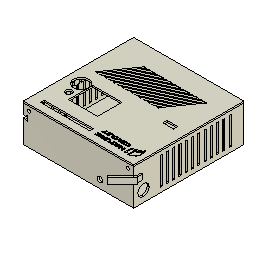
Focus maintainer v24 (Autodesk Fusion 360 design; units mm, degrees)
Autodesk Fusion 360 part; units mm, degrees
sketch "Sketch1" plane through (0, 0, 0) normal (0, 0, 1) x (1, 0, 0)
  line L0 (0, 0) -> (104, 0)
  line L1 (104, 0) -> (104, 104)
  line L2 (104, 104) -> (0, 104)
  line L3 (0, 104) -> (0, 0)
  line L4 (102.2, 1.8) -> (102.2, 102.2)
  line L5 (102.2, 102.2) -> (1.8, 102.2)
  line L6 (1.8, 102.2) -> (1.8, 1.8)
  line L7 (1.8, 1.8) -> (102.2, 1.8)
  dimension "d1" = 104
  dimension "d2" = 104
  dimension "d3" = -1.8
  constraint horizontal L0
  constraint vertical L1
  constraint horizontal L2
  constraint vertical L3
  constraint coincident L0.start L3.end
  measures "d1" distance of L0.start L0.end
  measures "d2" distance of L0.start L2.end
extrude "Extrude1" add sketch "Sketch1" against normal blind 1.5 contours L0 L1 L2 L3 | L4 L5 L6 L7 makes body 1
extrude "Extrude2" add sketch "Sketch1" along normal blind 32.5 bodies 1
hole "Hole1" at (5.5, 0, 28.5) direction (0, 1, 0) diameter 3 depth 105 tip angle 118 bodies 1
pattern_linear "R-Pattern1" count 2 spacing 93 along (1, 0, 0) of "Hole1"
sketch "Sketch2" plane through (0, 0, 0) normal (0, 0, 1) x (1, 0, 0)
  line L0 (0, 0) -> (104, 0)
  line L1 (104, 0) -> (104, 104)
  line L2 (104, 104) -> (0, 104)
  line L3 (0, 104) -> (0, 0)
  line L4 (102, 2) -> (102, 102)
  line L5 (102, 102) -> (2, 102)
  line L6 (2, 102) -> (2, 2)
  line L7 (2, 2) -> (102, 2)
  line L8 (100, 4) -> (100, 100)
  line L9 (100, 100) -> (4, 100)
  line L10 (4, 100) -> (4, 4)
  line L11 (4, 4) -> (100, 4)
  dimension "d17" = 104
  dimension "d18" = 104
  dimension "d19" = -2
  dimension "d20" = -4
  constraint horizontal L0
  constraint vertical L1
  constraint horizontal L2
  constraint vertical L3
  constraint coincident L0.start L3.end
  measures "d17" distance of L0.start L0.end
  measures "d18" distance of L0.start L2.end
extrude "Extrude3" add sketch "Sketch1" sketch "Sketch2" against normal blind 1.5 separate body contours L0 L1 L2 L3 | L4 L5 L6 L7 of sketch 2 contours L0 L1 L2 L3 | L4 L5 L6 L7 | L8 L9 L10 L11 makes body 2
extrude "Extrude4" add sketch "Sketch2" along normal blind 6.5 contours L4 L5 L6 L7 bodies 2
hole "Hole2" at (5.5, 2, 4.1) direction (0, 1, 0) diameter 3 depth 110 tip angle 118 bodies 2
pattern_linear "R-Pattern2" count 2 spacing 93 along (1, 0, 0) of "Hole2"
sketch "Sketch3" plane through (0, 0, 0) normal (0, 0, 1) x (1, 0, 0)
  line L0 (20, 81.5) -> (47.5, 81.5)
  line L1 (47.5, 81.5) -> (47.5, 58.5)
  line L2 (47.5, 58.5) -> (20, 58.5)
  line L3 (20, 58.5) -> (20, 81.5)
  line L4 (100, 100) -> (4, 100)
  line L5 (100, 4) -> (100, 100)
  circle A0 centre (12.9, 62.5) radius 7.1
  line L6 (9, 97) -> (55.5, 97)
  line L7 (55.5, 97) -> (55.5, 93.5)
  line L8 (55.5, 93.5) -> (9, 93.5)
  line L9 (9, 93.5) -> (9, 97)
  circle A1 centre (14, 75) radius 3
  line L10 (4, 4) -> (4, 100)
  line L11 (83.5, 56) -> (93.5, 56)
  line L12 (93.5, 56) -> (93.5, 52)
  line L13 (93.5, 52) -> (83.5, 52)
  line L14 (83.5, 52) -> (83.5, 56)
  line L15 (31, 19) -> (29, 19)
  line L16 (29, 19) -> (10.072, 46.032)
  line L17 (31, 19) -> (12.0419, 46.032)
  line L18 (12.0419, 46.032) -> (10.072, 46.032)
  line L19 (35.0714, 19) -> (33.0714, 19)
  line L20 (33.0714, 19) -> (14.1434, 46.032)
  line L21 (35.0714, 19) -> (16.1133, 46.032)
  line L22 (16.1133, 46.032) -> (14.1434, 46.032)
  line L23 (39.1429, 19) -> (37.1429, 19)
  line L24 (37.1429, 19) -> (18.2148, 46.032)
  line L25 (39.1429, 19) -> (20.1847, 46.032)
  line L26 (20.1847, 46.032) -> (18.2148, 46.032)
  line L27 (43.2143, 19) -> (41.2143, 19)
  line L28 (41.2143, 19) -> (22.2863, 46.032)
  line L29 (43.2143, 19) -> (24.2561, 46.032)
  line L30 (24.2561, 46.032) -> (22.2863, 46.032)
  line L31 (47.2857, 19) -> (45.2857, 19)
  line L32 (45.2857, 19) -> (26.3577, 46.032)
  line L33 (47.2857, 19) -> (28.3276, 46.032)
  line L34 (28.3276, 46.032) -> (26.3577, 46.032)
  line L35 (51.3571, 19) -> (49.3571, 19)
  line L36 (49.3571, 19) -> (30.4291, 46.032)
  line L37 (51.3571, 19) -> (32.399, 46.032)
  line L38 (32.399, 46.032) -> (30.4291, 46.032)
  line L39 (55.4286, 19) -> (53.4286, 19)
  line L40 (53.4286, 19) -> (34.5005, 46.032)
  line L41 (55.4286, 19) -> (36.4704, 46.032)
  line L42 (36.4704, 46.032) -> (34.5005, 46.032)
  line L43 (59.5, 19) -> (57.5, 19)
  line L44 (57.5, 19) -> (38.572, 46.032)
  line L45 (59.5, 19) -> (40.5419, 46.032)
  line L46 (40.5419, 46.032) -> (38.572, 46.032)
  line L47 (63.5714, 19) -> (61.5714, 19)
  line L48 (61.5714, 19) -> (42.6434, 46.032)
  line L49 (63.5714, 19) -> (44.6133, 46.032)
  line L50 (44.6133, 46.032) -> (42.6434, 46.032)
  line L51 (67.6429, 19) -> (65.6429, 19)
  line L52 (65.6429, 19) -> (46.7148, 46.032)
  line L53 (67.6429, 19) -> (48.6847, 46.032)
  line L54 (48.6847, 46.032) -> (46.7148, 46.032)
  line L55 (71.7143, 19) -> (69.7143, 19)
  line L56 (69.7143, 19) -> (50.7863, 46.032)
  line L57 (71.7143, 19) -> (52.7561, 46.032)
  line L58 (52.7561, 46.032) -> (50.7863, 46.032)
  line L59 (75.7857, 19) -> (73.7857, 19)
  line L60 (73.7857, 19) -> (54.8577, 46.032)
  line L61 (75.7857, 19) -> (56.8276, 46.032)
  line L62 (56.8276, 46.032) -> (54.8577, 46.032)
  line L63 (79.8571, 19) -> (77.8571, 19)
  line L64 (77.8571, 19) -> (58.9291, 46.032)
  line L65 (79.8571, 19) -> (60.899, 46.032)
  line L66 (60.899, 46.032) -> (58.9291, 46.032)
  line L67 (83.9286, 19) -> (81.9286, 19)
  line L68 (81.9286, 19) -> (63.0005, 46.032)
  line L69 (83.9286, 19) -> (64.9704, 46.032)
  line L70 (64.9704, 46.032) -> (63.0005, 46.032)
  line L71 (88, 19) -> (86, 19)
  line L72 (86, 19) -> (67.072, 46.032)
  line L73 (88, 19) -> (69.0419, 46.032)
  line L74 (69.0419, 46.032) -> (67.072, 46.032)
  dimension "d34" = 18.5
  dimension "d36" = 27.5
  dimension "d37" = 23
  dimension "d38" = 14.2
  dimension "d39" = 19
  dimension "d41" = 3
  dimension "d42" = 46.5
  dimension "d43" = 3.5
  dimension "d44" = 6
  dimension "d45" = 25
  dimension "d48" = 16
  dimension "d50" = 7.1
  dimension "d51" = 10
  dimension "d52" = 5
  dimension "d53" = 44
  dimension "d54" = 6.5
  dimension "d55" = 10
  dimension "d56" = 4
  dimension "d63" = 33
  dimension "d68" = 15
  dimension "d71" = 57
  dimension "d72" = 0
  constraint horizontal L0
  constraint vertical L1
  constraint horizontal L2
  constraint vertical L3
  constraint horizontal L6
  constraint vertical L7
  constraint horizontal L8
  constraint vertical L9
  constraint horizontal L11
  constraint vertical L12
  constraint horizontal L13
  constraint vertical L14
  constraint horizontal L15
  constraint parallel L15 L18
  measures "d34" distance of L0.end L4
  measures "d36" distance of L0.start L0.end
  measures "d37" distance of L0.start L2.end
  measures "d38" diameter of A0
  measures "d39" vertical distance of L0.end A0.centre
  measures "d41" distance of L4 L6.end
  measures "d42" distance of L7.end L8.end
  measures "d43" distance of L6.start L8.end
  measures "d44" diameter of A1
  measures "d45" vertical distance of L4.start A1.centre
  measures "d48" horizontal distance of L0.start L4.end
  measures "d50" horizontal distance of L2.end A0.centre
  measures "d51" distance of A1.centre L10
  measures "d52" horizontal distance of L6.start L4.end
  measures "d53" vertical distance of L4.start L11.end
  measures "d54" horizontal distance of L4.start L11.end
  measures "d55" distance of L12.end L13.end
  measures "d56" distance of L11.start L13.end
  measures "d63" distance of L15.end L16.end
  measures "d68" distance of L10.start L15
extrude "Extrude5" cut sketch "Sketch3" against normal blind 1.5 bodies 2
sketch "Sketch4" plane through (102.2, 0, 0) normal (-1, 0, 0) x (0, -1, 0)
  line L0 (-102.2, 0) -> (-1.8, 0)
  line L1 (-1.8, 0) -> (-1.8, 32.5)
  line L2 (-1.8, 32.5) -> (-102.2, 32.5)
  line L3 (-102.2, 32.5) -> (-102.2, 0)
  line L4 (-6.8, 3.5) -> (-10.8544, 3.5)
  line L5 (-4.05, 3.5) -> (-14.55, 3.5)
  line L6 (-14.55, 3.5) -> (-14.55, 14)
  line L7 (-14.55, 14) -> (-4.05, 14)
  line L8 (-4.05, 14) -> (-4.05, 3.5)
  dimension "d86" = 10.5
  dimension "d87" = 10.5
  dimension "d88" = 2.25
  dimension "d89" = 3.5
  constraint horizontal L4
  constraint horizontal L5
  constraint vertical L6
  constraint horizontal L7
  constraint vertical L8
  measures "d86" distance of L5.start L5.end
  measures "d87" distance of L5.start L7.end
  measures "d88" distance of L1 L5.start
  measures "d89" distance of L0 L5
sketch "Sketch5" plane through (0, 1.8, 0) normal (0, 1, 0) x (-1, 0, 0)
  circle A0 centre (-98.5, 28.5) radius 1.5
  circle A1 centre (-5.5, 28.5) radius 1.5
  line L0 (-102.2, 0) -> (-1.8, 0)
  line L1 (-1.8, 0) -> (-1.8, 32.5)
  line L2 (-1.8, 32.5) -> (-102.2, 32.5)
  line L3 (-102.2, 32.5) -> (-102.2, 0)
  circle A2 centre (-72.2, 6) radius 2.5
  dimension "d79" = 5
  dimension "d80" = 30
  dimension "d81" = 6
  measures "d79" diameter of A2
  measures "d80" distance of L3 A2.centre
  measures "d81" distance of L0 A2.centre
extrude "Extrude7" cut sketch "Sketch5" against normal blind 6 contours A2 bodies 1
extrude "Extrude8" cut sketch "Sketch4" against normal blind 2 contours L4 L5 L6 L7 L8 bodies 1
fillet "Fillet1" radius 5 4 edges at (103.1, 4.05, 14) (103.1, 14.55, 14) (103.1, 14.55, 3.5) (103.1, 4.05, 3.5) on bodies 1
sketch "Sketch6" plane through (0, 0, 0) normal (0, -1, 0) x (1, 0, 0)
  circle A0 centre (72.2, 6) radius 2.5
  circle A1 centre (98.5, 28.5) radius 1.5
  circle A2 centre (5.5, 28.5) radius 1.5
  line L0 (0, 32.5) -> (0, -1.5)
  line L1 (0, -1.5) -> (104, -1.5)
  line L2 (104, -1.5) -> (104, 32.5)
  line L3 (104, 32.5) -> (0, 32.5)
  line L4 (104, 22.7437) -> (102, 22.7437)
  line L5 (102, 22.7437) -> (100.4679, 24.0293)
  line L6 (100.4679, 24.0293) -> (100.4679, 19.0293)
  line L7 (100.4679, 19.0293) -> (102, 20.3149)
  line L8 (100.4679, 19.0293) -> (102.4679, 19.0293) construction
  line L9 (102, 20.3149) -> (104, 20.3149)
  line L10 (104, 20.3149) -> (104, 22.7437)
  line L11 (52, -1.5) -> (52, 32.5)
  line L12 (2, 22.7437) -> (3.5321, 24.0293)
  line L13 (3.5321, 24.0293) -> (3.5321, 19.0293)
  line L14 (3.5321, 19.0293) -> (1.5321, 19.0293) construction
  line L15 (3.5321, 19.0293) -> (2, 20.3149)
  line L16 (0, 22.7437) -> (2, 22.7437)
  line L17 (2, 20.3149) -> (0, 20.3149)
  line L18 (104, 22.7437) -> (104.2, 22.7437)
  line L19 (104.2, 22.7437) -> (104.2, 23.9437)
  line L20 (104.2, 23.9437) -> (105.7, 23.9437)
  line L21 (104, 20.3149) -> (104.2, 20.3149)
  line L22 (104.2, 20.3149) -> (104.2, 19.1149)
  line L23 (104.2, 19.1149) -> (105.7, 19.1149)
  line L24 (105.7, 19.1149) -> (105.7, 23.9437)
  dimension "d92" = 2
  dimension "d93" = 140
  dimension "d94" = 2
  dimension "d95" = 5
  dimension "d96" = 2
  dimension "d97" = 40
  dimension "d129" = 0.2
  dimension "d130" = 1.2
  dimension "d131" = 1.5
  dimension "d132" = 0.2
  dimension "d133" = 1.2
  dimension "d134" = 1.5
  constraint coincident L2 L4.start
  constraint perpendicular L2 L4
  constraint vertical L6
  constraint horizontal L8
  constraint coincident L2 L9.end
  constraint perpendicular L2 L9
  constraint midpoint L1 L11.start
  constraint midpoint L3 L11.end
  constraint symmetric L4.start L11 L16.start
  constraint symmetric L4.end L11 L12.start
  constraint symmetric L5.end L11 L12.end
  constraint symmetric L6.end L11 L13.end
  constraint symmetric L7.end L11 L15.end
  constraint symmetric L8.end L11 L14.end
  constraint symmetric L9.end L11 L17.end
  constraint perpendicular L2 L18
  constraint perpendicular L4 L19
  constraint perpendicular L19 L20
  constraint perpendicular L2 L21
  constraint perpendicular L21 L22
  constraint perpendicular L22 L23
  measures "d92" distance of L4.start L4.end
  measures "d93" angle of L4 L5
  measures "d94" distance of L4.end L5.end
  measures "d95" distance of L5.end L6.end
  measures "d96" distance of L6.end L7.end
  measures "d97" angle of L7 L8
  measures "d129" distance of L4.start L18.end
  measures "d130" distance of L18.end L19.end
  measures "d131" distance of L19.end L20.end
  measures "d132" distance of L9.end L21.end
  measures "d133" distance of L21.end L22.end
  measures "d134" distance of L22.end L23.end
extrude "Extrude9" cut sketch "Sketch6" against normal blind 7 contours L0 L12 L13 L15 L16 L17 | L2 L4 L5 L6 L7 L9 L10 bodies 1
extrude "Extrude10" add sketch "Sketch6" along normal blind -7 and the other way blind -8 separate body contours L2 L10 L18 L19 L20 L21 L22 L23 L24 | L2 L4 L5 L6 L7 L9 L10 makes body 3
ref_plane "WorkPlane1" through (104, 0, 21.5293) normal (-0.707107, 0.707107, 0) x (0, 0, 1)
sketch "Sketch7" plane through (52, -52, 0) normal (-0.707107, 0.707107, 0) x (0, 0, 1)
  line L0 (19, 76) -> (24.9317, 76)
  line L1 (24.9317, 76) -> (24.9317, 56)
  line L2 (24.9317, 56) -> (19, 56)
  line L3 (19, 56) -> (19, 76)
  dimension "d105" = 20
  constraint horizontal L0
  constraint vertical L1
  constraint horizontal L2
  constraint vertical L3
  measures "d105" distance of L0.start L2.end
extrude "Extrude11" cut sketch "Sketch7" against normal blind 8 bodies 3
extrude "Extrude12" add sketch "Sketch7" against normal blind 2 bodies 3
move_face "OffsetFaces1" offset -0.2 5 faces at (102.7333, 1.7333, 22.7437) (100.9786, 0.4893, 23.6008) (100.4679, -0.0214, 22.3626) (100.9786, 0.4893, 19.4578) (102.7333, 1.7333, 20.3149) on bodies 3
sketch "Sketch8" plane through (0, 0, 0) normal (-1, 0, 0) x (0, -1, 0)
  line L0 (-7, 22.7437) -> (0, 22.7437)
  line L1 (0, 22.7437) -> (0, 32.5)
  line L2 (0, 32.5) -> (-104, 32.5)
  line L3 (-104, 32.5) -> (-104, -1.5)
  line L4 (-104, -1.5) -> (0, -1.5)
  line L5 (0, -1.5) -> (0, 20.3149)
  line L6 (0, 20.3149) -> (-7, 20.3149)
  line L7 (-7, 20.3149) -> (-7, 22.7437)
  line L8 (-92, 29) -> (-90, 29)
  line L9 (-90, 29) -> (-90, 3)
  line L10 (-90, 3) -> (-92, 3)
  line L11 (-92, 3) -> (-92, 29)
  constraint horizontal L8
  constraint vertical L9
  constraint horizontal L10
  constraint vertical L11
extrude "Extrude13" cut sketch "Sketch8" against normal blind 120 contours L8 L9 L10 L11 bodies 1
pattern_linear "R-Pattern3" count 12 spacing 5.9091 along (0, -1, 0) of "Extrude13"
sketch "Sketch9" plane through (0, 0, -1.5) normal (0, 0, -1) x (1, 0, 0)
  line L0 (60.899, -46.032) -> (58.9291, -46.032)
  line L1 (58.9291, -46.032) -> (77.8571, -19)
  line L2 (77.8571, -19) -> (79.8571, -19)
  line L3 (79.8571, -19) -> (60.899, -46.032)
  line L4 (44.6133, -46.032) -> (42.6434, -46.032)
  line L5 (42.6434, -46.032) -> (61.5714, -19)
  line L6 (61.5714, -19) -> (63.5714, -19)
  line L7 (63.5714, -19) -> (44.6133, -46.032)
  line L8 (28.3276, -46.032) -> (26.3577, -46.032)
  line L9 (26.3577, -46.032) -> (45.2857, -19)
  line L10 (45.2857, -19) -> (47.2857, -19)
  line L11 (47.2857, -19) -> (28.3276, -46.032)
  line L12 (12.0419, -46.032) -> (10.072, -46.032)
  line L13 (10.072, -46.032) -> (29, -19)
  line L14 (29, -19) -> (31, -19)
  line L15 (31, -19) -> (12.0419, -46.032)
  circle A0 centre (14, -75) radius 3
  line L16 (16.1133, -46.032) -> (14.1434, -46.032)
  line L17 (14.1434, -46.032) -> (33.0714, -19)
  line L18 (33.0714, -19) -> (35.0714, -19)
  line L19 (35.0714, -19) -> (16.1133, -46.032)
  line L20 (32.399, -46.032) -> (30.4291, -46.032)
  line L21 (30.4291, -46.032) -> (49.3571, -19)
  line L22 (49.3571, -19) -> (51.3571, -19)
  line L23 (51.3571, -19) -> (32.399, -46.032)
  line L24 (48.6847, -46.032) -> (46.7148, -46.032)
  line L25 (46.7148, -46.032) -> (65.6429, -19)
  line L26 (65.6429, -19) -> (67.6429, -19)
  line L27 (67.6429, -19) -> (48.6847, -46.032)
  line L28 (64.9704, -46.032) -> (63.0005, -46.032)
  line L29 (63.0005, -46.032) -> (81.9286, -19)
  line L30 (81.9286, -19) -> (83.9286, -19)
  line L31 (83.9286, -19) -> (64.9704, -46.032)
  line L32 (56.8276, -46.032) -> (54.8577, -46.032)
  line L33 (54.8577, -46.032) -> (73.7857, -19)
  line L34 (73.7857, -19) -> (75.7857, -19)
  line L35 (75.7857, -19) -> (56.8276, -46.032)
  line L36 (40.5419, -46.032) -> (38.572, -46.032)
  line L37 (38.572, -46.032) -> (57.5, -19)
  line L38 (57.5, -19) -> (59.5, -19)
  line L39 (59.5, -19) -> (40.5419, -46.032)
  line L40 (24.2561, -46.032) -> (22.2863, -46.032)
  line L41 (22.2863, -46.032) -> (41.2143, -19)
  line L42 (41.2143, -19) -> (43.2143, -19)
  line L43 (43.2143, -19) -> (24.2561, -46.032)
  line L44 (93.5, -52) -> (93.5, -56)
  line L45 (93.5, -56) -> (83.5, -56)
  line L46 (83.5, -56) -> (83.5, -52)
  line L47 (83.5, -52) -> (93.5, -52)
  line L48 (47.5, -58.5) -> (47.5, -81.5)
  line L49 (47.5, -81.5) -> (20, -81.5)
  line L50 (20, -81.5) -> (20, -62.5)
  circle A1 centre (12.9, -62.5) radius 7.1
  line L51 (20, -62.5) -> (20, -58.5)
  line L52 (20, -58.5) -> (47.5, -58.5)
  line L53 (55.5, -93.5) -> (55.5, -97)
  line L54 (55.5, -97) -> (9, -97)
  line L55 (9, -97) -> (9, -93.5)
  line L56 (9, -93.5) -> (55.5, -93.5)
  line L57 (20.1847, -46.032) -> (18.2148, -46.032)
  line L58 (18.2148, -46.032) -> (37.1429, -19)
  line L59 (37.1429, -19) -> (39.1429, -19)
  line L60 (39.1429, -19) -> (20.1847, -46.032)
  line L61 (36.4704, -46.032) -> (34.5005, -46.032)
  line L62 (34.5005, -46.032) -> (53.4286, -19)
  line L63 (53.4286, -19) -> (55.4286, -19)
  line L64 (55.4286, -19) -> (36.4704, -46.032)
  line L65 (52.7561, -46.032) -> (50.7863, -46.032)
  line L66 (50.7863, -46.032) -> (69.7143, -19)
  line L67 (69.7143, -19) -> (71.7143, -19)
  line L68 (71.7143, -19) -> (52.7561, -46.032)
  line L69 (69.0419, -46.032) -> (67.072, -46.032)
  line L70 (67.072, -46.032) -> (86, -19)
  line L71 (86, -19) -> (88, -19)
  line L72 (88, -19) -> (69.0419, -46.032)
  line L73 (0, 0) -> (0, -104)
  line L74 (0, -104) -> (104, -104)
  line L75 (104, -104) -> (104, 0)
  line L76 (104, 0) -> (0, 0)
  spline S0 degree 3 poles (98.7844, -87.4951) (99.1077, -88.4839) (99.0819, -89.3983) (99.0819, -90.4193) knots 0 0 0 0 1 1 1 1
  spline S1 degree 3 poles (99.0819, -90.4193) (99.0819, -92.0513) (99.3129, -93.8226) (98.2772, -95.2143) knots 0 0 0 0 1 1 1 1
  spline S2 degree 3 poles (98.2772, -95.2143) (97.4381, -96.3429) (95.5453, -97.168) (94.2868, -97.8019) knots 0 0 0 0 1 1 1 1
  line L77 (94.2868, -97.8019) -> (92.7057, -98.6644)
  line L78 (92.7057, -98.6644) -> (92.7057, -97.8457)
  line L79 (92.7057, -97.8457) -> (92.6495, -97.144)
  line L80 (92.6495, -97.144) -> (92.6495, -96.957)
  line L81 (92.6495, -96.957) -> (92.6495, -96.5105)
  line L82 (92.6495, -96.5105) -> (92.6495, -94.9219)
  spline S3 degree 3 poles (92.6495, -94.9219) (92.6495, -94.0261) (92.6103, -93.2367) (93.1635, -92.4659) knots 0 0 0 0 1 1 1 1
  spline S4 degree 3 poles (93.1635, -92.4659) (93.5115, -91.9806) (94.0021, -91.7169) (94.5207, -91.4572) knots 0 0 0 0 1 1 1 1
  spline S5 degree 3 poles (94.5207, -91.4572) (95.4932, -90.9713) (96.7762, -90.6432) (97.62, -89.9795) knots 0 0 0 0 1 1 1 1
  spline S6 degree 3 poles (97.62, -89.9795) (98.1006, -89.6018) (98.4831, -89.1381) (98.6603, -88.548) knots 0 0 0 0 1 1 1 1
  line L83 (98.6603, -88.548) -> (98.7844, -87.4951)
  spline S7 degree 3 poles (89.3158, -98.1858) (89.2071, -97.9116) (89.2573, -97.0104) (89.2573, -96.6654) knots 0 0 0 0 1 1 1 1
  line L84 (89.2573, -96.6654) -> (89.2573, -93.8586)
  spline S8 degree 3 poles (89.2573, -93.8586) (89.2573, -93.1575) (89.1597, -92.7107) (89.6041, -92.1043) knots 0 0 0 0 1 1 1 1
  spline S9 degree 3 poles (89.6041, -92.1043) (90.2228, -91.2599) (91.7285, -90.6968) (92.7074, -90.3693) knots 0 0 0 0 1 1 1 1
  spline S10 degree 3 poles (92.7074, -90.3693) (93.957, -89.9512) (95.223, -89.5799) (96.3914, -88.9595) knots 0 0 0 0 1 1 1 1
  spline S11 degree 3 poles (96.3914, -88.9595) (97.4907, -88.3759) (98.0825, -87.7104) (97.8533, -86.4322) knots 0 0 0 0 1 1 1 1
  spline S12 degree 3 poles (97.8533, -86.4322) (98.2486, -86.6444) (98.745, -87.207) (98.8316, -87.6602) knots 0 0 0 0 1 1 1 1
  spline S13 degree 3 poles (98.8316, -87.6602) (98.9433, -88.2438) (98.5737, -89.0998) (98.1936, -89.5314) knots 0 0 0 0 1 1 1 1
  spline S14 degree 3 poles (98.1936, -89.5314) (96.9879, -90.9015) (94.6237, -90.998) (93.4144, -92.2803) knots 0 0 0 0 1 1 1 1
  spline S15 degree 3 poles (93.4144, -92.2803) (92.4829, -93.2686) (92.7097, -94.8188) (92.7074, -96.0807) knots 0 0 0 0 1 1 1 1
  spline S16 degree 3 poles (92.7074, -96.0807) (92.7074, -96.2035) (92.7221, -96.4087) (92.6495, -96.5105) knots 0 0 0 0 1 1 1 1
  spline S17 degree 3 poles (92.6495, -96.5105) (92.5583, -96.638) (91.9496, -96.8391) (91.7718, -96.9111) knots 0 0 0 0 1 1 1 1
  spline S18 degree 3 poles (91.7718, -96.9111) (90.9941, -97.2245) (89.9737, -97.6783) (89.3158, -98.1858) knots 0 0 0 0 1 1 1 1
  line L85 (86.7727, -97.3774) -> (86.2481, -97.3774)
  spline S19 degree 2 poles (86.2481, -97.3774) (85.9825, -97.3774) (85.7363, -97.1526) knots 0 0 0 1 1 1
  line L86 (85.7363, -97.1526) -> (83.7383, -95.5315)
  line L87 (83.7383, -95.5315) -> (83.7383, -97.0241)
  spline S20 degree 2 poles (83.7383, -97.0241) (83.7383, -97.2618) (83.4877, -97.3646) knots 0 0 0 1 1 1
  spline S21 degree 2 poles (83.4877, -97.3646) (83.4385, -97.3774) (83.3935, -97.3774) knots 0 0 0 1 1 1
  line L88 (83.3935, -97.3774) -> (82.8196, -97.3774)
  line L89 (82.8196, -97.3774) -> (82.8196, -94.3066)
  line L90 (82.8196, -94.3066) -> (83.3443, -94.3066)
  spline S22 degree 2 poles (83.3443, -94.3066) (83.6162, -94.3066) (83.8903, -94.5614) knots 0 0 0 1 1 1
  spline S23 degree 2 poles (83.8903, -94.5614) (83.8925, -94.5635) (84.0124, -94.6578) knots 0 0 0 1 1 1
  spline S24 degree 2 poles (84.0124, -94.6578) (84.1302, -94.752) (84.3721, -94.9447) knots 0 0 0 1 1 1
  spline S25 degree 2 poles (84.3721, -94.9447) (84.612, -95.1374) (84.9803, -95.4308) knots 0 0 0 1 1 1
  spline S26 degree 2 poles (84.9803, -95.4308) (85.3487, -95.7242) (85.8498, -96.1268) knots 0 0 0 1 1 1
  line L91 (85.8498, -96.1268) -> (85.854, -96.1268)
  line L92 (85.854, -96.1268) -> (85.854, -94.3066)
  line L93 (85.854, -94.3066) -> (86.7727, -94.3066)
  line L94 (86.7727, -94.3066) -> (86.7727, -97.3774)
  spline S27 degree 2 poles (80.3805, -94.4608) (80.3805, -94.5871) (80.3291, -94.7006) knots 0 0 0 1 1 1
  spline S28 degree 2 poles (80.3291, -94.7006) (80.2755, -94.8162) (80.1813, -94.904) knots 0 0 0 1 1 1
  spline S29 degree 2 poles (80.1813, -94.904) (80.0871, -94.994) (79.9586, -95.0454) knots 0 0 0 1 1 1
  spline S30 degree 2 poles (79.9586, -95.0454) (79.828, -95.0989) (79.6738, -95.0989) knots 0 0 0 1 1 1
  line L95 (79.6738, -95.0989) -> (78.9928, -95.0989)
  line L96 (78.9928, -95.0989) -> (79.8644, -96.5144)
  line L97 (79.8644, -96.5144) -> (81.2349, -94.2959)
  spline S31 degree 2 poles (81.2349, -94.2959) (82.2842, -94.2959) (82.2842, -94.298) knots 0 0 0 1 1 1
  spline S32 degree 2 poles (82.2842, -94.298) (82.2543, -94.3451) (82.1814, -94.4608) knots 0 0 0 1 1 1
  spline S33 degree 2 poles (82.1814, -94.4608) (82.1086, -94.5785) (82.0037, -94.7477) knots 0 0 0 1 1 1
  spline S34 degree 2 poles (82.0037, -94.7477) (81.8988, -94.9169) (81.7681, -95.1289) knots 0 0 0 1 1 1
  spline S35 degree 2 poles (81.7681, -95.1289) (81.6375, -95.343) (81.4919, -95.5807) knots 0 0 0 1 1 1
  spline S36 degree 2 poles (81.4919, -95.5807) (81.3441, -95.8184) (81.1878, -96.0711) knots 0 0 0 1 1 1
  spline S37 degree 2 poles (81.1878, -96.0711) (81.0315, -96.3238) (80.8773, -96.5744) knots 0 0 0 1 1 1
  spline S38 degree 2 poles (80.8773, -96.5744) (80.8023, -96.6986) (80.7424, -96.7949) knots 0 0 0 1 1 1
  spline S39 degree 2 poles (80.7424, -96.7949) (80.6824, -96.8934) (80.631, -96.9663) knots 0 0 0 1 1 1
  spline S40 degree 2 poles (80.631, -96.9663) (80.5796, -97.0391) (80.5368, -97.0883) knots 0 0 0 1 1 1
  spline S41 degree 2 poles (80.5368, -97.0883) (80.4918, -97.1397) (80.449, -97.1675) knots 0 0 0 1 1 1
  spline S42 degree 2 poles (80.449, -97.1675) (80.3077, -97.2768) (80.1621, -97.3217) knots 0 0 0 1 1 1
  spline S43 degree 2 poles (80.1621, -97.3217) (80.0143, -97.3667) (79.8323, -97.3667) knots 0 0 0 1 1 1
  spline S44 degree 2 poles (79.8323, -97.3667) (79.6781, -97.3667) (79.5132, -97.3003) knots 0 0 0 1 1 1
  spline S45 degree 2 poles (79.5132, -97.3003) (79.3483, -97.2339) (79.1813, -97.0669) knots 0 0 0 1 1 1
  spline S46 degree 2 poles (79.1813, -97.0669) (79.0935, -96.9705) (79.0571, -96.9063) knots 0 0 0 1 1 1
  line L98 (79.0571, -96.9063) -> (77.4467, -94.2959)
  line L99 (77.4467, -94.2959) -> (80.3783, -94.2959)
  line L100 (80.3783, -94.2959) -> (80.3805, -94.4608)
  line L101 (76.6329, -96.5422) -> (78.0506, -96.5422)
  line L102 (78.0506, -96.5422) -> (78.0506, -96.6729)
  spline S47 degree 2 poles (78.0506, -96.6729) (78.0506, -96.8977) (77.8536, -97.1333) knots 0 0 0 1 1 1
  spline S48 degree 2 poles (77.8536, -97.1333) (77.6715, -97.3025) (77.5538, -97.326) knots 0 0 0 1 1 1
  spline S49 degree 2 poles (77.5538, -97.326) (77.4467, -97.3667) (77.3567, -97.3667) knots 0 0 0 1 1 1
  line L103 (77.3567, -97.3667) -> (74.2859, -97.3667)
  line L104 (74.2859, -97.3667) -> (74.2859, -97.2404)
  spline S50 degree 2 poles (74.2859, -97.2404) (74.2859, -97.0134) (74.4786, -96.7842) knots 0 0 0 1 1 1
  spline S51 degree 2 poles (74.4786, -96.7842) (74.6757, -96.5422) (75.1146, -96.5422) knots 0 0 0 1 1 1
  line L105 (75.1146, -96.5422) -> (75.71, -96.5422)
  line L106 (75.71, -96.5422) -> (75.71, -94.2959)
  line L107 (75.71, -94.2959) -> (76.6329, -94.2959)
  line L108 (76.6329, -94.2959) -> (76.6329, -96.5422)
  spline S52 degree 2 poles (73.7505, -96.9877) (73.7505, -97.2318) (73.4764, -97.3517) knots 0 0 0 1 1 1
  spline S53 degree 2 poles (73.4764, -97.3517) (73.4293, -97.3667) (73.3715, -97.3667) knots 0 0 0 1 1 1
  line L109 (73.3715, -97.3667) -> (72.8554, -97.3667)
  line L110 (72.8554, -97.3667) -> (72.8554, -95.8377)
  spline S54 degree 2 poles (72.8554, -95.8377) (72.8554, -95.7049) (72.8147, -95.5979) knots 0 0 0 1 1 1
  spline S55 degree 2 poles (72.8147, -95.5979) (72.7719, -95.4908) (72.7012, -95.4094) knots 0 0 0 1 1 1
  spline S56 degree 2 poles (72.7012, -95.4094) (72.6284, -95.328) (72.5321, -95.2681) knots 0 0 0 1 1 1
  spline S57 degree 2 poles (72.5321, -95.2681) (72.4335, -95.2102) (72.3243, -95.1717) knots 0 0 0 1 1 1
  spline S58 degree 2 poles (72.3243, -95.1717) (72.213, -95.1353) (72.0952, -95.1182) knots 0 0 0 1 1 1
  spline S59 degree 2 poles (72.0952, -95.1182) (71.9774, -95.101) (71.8639, -95.101) knots 0 0 0 1 1 1
  spline S60 degree 2 poles (71.8639, -95.101) (71.3992, -95.101) (71.0523, -95.3516) knots 0 0 0 1 1 1
  spline S61 degree 2 poles (71.0523, -95.3516) (70.8125, -95.5572) (70.8125, -95.8099) knots 0 0 0 1 1 1
  line L111 (70.8125, -95.8099) -> (70.8125, -96.8699)
  spline S62 degree 2 poles (70.8125, -96.8699) (70.8125, -97.1354) (70.6947, -97.2339) knots 0 0 0 1 1 1
  spline S63 degree 2 poles (70.6947, -97.2339) (70.5769, -97.3517) (70.4056, -97.3517) knots 0 0 0 1 1 1
  line L112 (70.4056, -97.3517) -> (69.8981, -97.3517)
  line L113 (69.8981, -97.3517) -> (69.8981, -95.7542)
  spline S64 degree 2 poles (69.8981, -95.7542) (69.8981, -95.0689) (70.5362, -94.6299) knots 0 0 0 1 1 1
  spline S65 degree 2 poles (70.5362, -94.6299) (71.0909, -94.2959) (71.7354, -94.2959) knots 0 0 0 1 1 1
  line L114 (71.7354, -94.2959) -> (71.8446, -94.2959)
  spline S66 degree 2 poles (71.8446, -94.2959) (72.5963, -94.2959) (73.2045, -94.7177) knots 0 0 0 1 1 1
  spline S67 degree 2 poles (73.2045, -94.7177) (73.7505, -95.1589) (73.7505, -95.7499) knots 0 0 0 1 1 1
  line L115 (73.7505, -95.7499) -> (73.7505, -96.9877)
  spline S68 degree 2 poles (69.2556, -95.4694) (69.2556, -95.6814) (69.095, -95.9148) knots 0 0 0 1 1 1
  spline S69 degree 2 poles (69.095, -95.9148) (68.8402, -96.2467) (68.4033, -96.2467) knots 0 0 0 1 1 1
  line L116 (68.4033, -96.2467) -> (68.3369, -96.2467)
  line L117 (68.3369, -96.2467) -> (68.3369, -95.797)
  line L118 (68.3369, -95.797) -> (66.5938, -95.797)
  spline S70 degree 2 poles (66.5938, -95.797) (66.4268, -95.797) (66.3261, -95.8848) knots 0 0 0 1 1 1
  spline S71 degree 2 poles (66.3261, -95.8848) (66.2255, -95.9748) (66.2255, -96.1418) knots 0 0 0 1 1 1
  line L119 (66.2255, -96.1418) -> (66.2255, -96.2018)
  spline S72 degree 2 poles (66.2255, -96.2018) (66.2255, -96.4523) (66.4589, -96.5294) knots 0 0 0 1 1 1
  spline S73 degree 2 poles (66.4589, -96.5294) (66.491, -96.5422) (66.5488, -96.5422) knots 0 0 0 1 1 1
  line L120 (66.5488, -96.5422) -> (68.3369, -96.5422)
  spline S74 degree 2 poles (68.3369, -96.5422) (68.7053, -96.5422) (68.8787, -96.6772) knots 0 0 0 1 1 1
  spline S75 degree 2 poles (68.8787, -96.6772) (68.9601, -96.7264) (69.0308, -96.7971) knots 0 0 0 1 1 1
  spline S76 degree 2 poles (69.0308, -96.7971) (69.0993, -96.8699) (69.1507, -96.9577) knots 0 0 0 1 1 1
  spline S77 degree 2 poles (69.1507, -96.9577) (69.2, -97.0476) (69.2278, -97.1504) knots 0 0 0 1 1 1
  spline S78 degree 2 poles (69.2278, -97.1504) (69.2556, -97.2553) (69.2556, -97.3667) knots 0 0 0 1 1 1
  line L121 (69.2556, -97.3667) -> (66.5381, -97.3667)
  spline S79 degree 2 poles (66.5381, -97.3667) (66.2747, -97.3667) (66.0499, -97.2832) knots 0 0 0 1 1 1
  spline S80 degree 2 poles (66.0499, -97.2832) (65.8229, -97.1997) (65.658, -97.0433) knots 0 0 0 1 1 1
  spline S81 degree 2 poles (65.658, -97.0433) (65.491, -96.887) (65.3967, -96.6622) knots 0 0 0 1 1 1
  spline S82 degree 2 poles (65.3967, -96.6622) (65.3025, -96.4373) (65.3025, -96.1568) knots 0 0 0 1 1 1
  spline S83 degree 2 poles (65.3025, -96.1568) (65.3025, -95.5165) (65.8357, -95.1653) knots 0 0 0 1 1 1
  line L122 (65.8357, -95.1653) -> (65.84, -95.1653)
  line L123 (65.84, -95.1653) -> (65.84, -95.161)
  line L124 (65.84, -95.161) -> (65.0113, -94.3002)
  line L125 (65.0113, -94.3002) -> (65.0113, -94.2959)
  line L126 (65.0113, -94.2959) -> (66.2255, -94.2959)
  line L127 (66.2255, -94.2959) -> (66.885, -94.9726)
  line L128 (66.885, -94.9726) -> (68.3369, -94.9726)
  line L129 (68.3369, -94.9726) -> (68.3369, -94.298)
  line L130 (68.3369, -94.298) -> (69.2556, -94.298)
  line L131 (69.2556, -94.298) -> (69.2556, -95.4694)
  spline S84 degree 2 poles (64.4759, -96.6729) (64.4759, -96.8977) (64.2789, -97.1333) knots 0 0 0 1 1 1
  spline S85 degree 2 poles (64.2789, -97.1333) (64.0969, -97.3025) (63.9791, -97.326) knots 0 0 0 1 1 1
  spline S86 degree 2 poles (63.9791, -97.326) (63.8763, -97.3667) (63.7821, -97.3667) knots 0 0 0 1 1 1
  line L132 (63.7821, -97.3667) -> (60.7112, -97.3667)
  line L133 (60.7112, -97.3667) -> (60.7112, -97.2404)
  spline S87 degree 2 poles (60.7112, -97.2404) (60.7112, -97.0498) (60.8547, -96.842) knots 0 0 0 1 1 1
  spline S88 degree 2 poles (60.8547, -96.842) (60.9275, -96.7521) (61.0003, -96.6943) knots 0 0 0 1 1 1
  spline S89 degree 2 poles (61.0003, -96.6943) (61.071, -96.6365) (61.1524, -96.6022) knots 0 0 0 1 1 1
  spline S90 degree 2 poles (61.1524, -96.6022) (61.2316, -96.5701) (61.3258, -96.5551) knots 0 0 0 1 1 1
  spline S91 degree 2 poles (61.3258, -96.5551) (61.4201, -96.5422) (61.5357, -96.5422) knots 0 0 0 1 1 1
  line L134 (61.5357, -96.5422) -> (64.4759, -96.5422)
  line L135 (64.4759, -96.5422) -> (64.4759, -96.6729)
  spline S92 degree 2 poles (64.4759, -95.4694) (64.4759, -95.7221) (64.2618, -95.9812) knots 0 0 0 1 1 1
  spline S93 degree 2 poles (64.2618, -95.9812) (64.0155, -96.2467) (63.6108, -96.2467) knots 0 0 0 1 1 1
  line L136 (63.6108, -96.2467) -> (61.3837, -96.2467)
  spline S94 degree 2 poles (61.3837, -96.2467) (61.3837, -96.039) (61.4372, -95.8891) knots 0 0 0 1 1 1
  spline S95 degree 2 poles (61.4372, -95.8891) (61.4907, -95.7413) (61.6064, -95.6321) knots 0 0 0 1 1 1
  spline S96 degree 2 poles (61.6064, -95.6321) (61.7691, -95.4822) (61.9297, -95.4437) knots 0 0 0 1 1 1
  spline S97 degree 2 poles (61.9297, -95.4437) (62.0197, -95.4158) (62.221, -95.4158) knots 0 0 0 1 1 1
  line L137 (62.221, -95.4158) -> (63.5572, -95.4158)
  line L138 (63.5572, -95.4158) -> (63.5572, -95.1203)
  line L139 (63.5572, -95.1203) -> (60.7112, -95.1203)
  line L140 (60.7112, -95.1203) -> (60.7112, -94.9897)
  spline S98 degree 2 poles (60.7112, -94.9897) (60.7112, -94.7648) (60.9082, -94.5293) knots 0 0 0 1 1 1
  spline S99 degree 2 poles (60.9082, -94.5293) (61.0903, -94.3601) (61.2081, -94.3365) knots 0 0 0 1 1 1
  spline S100 degree 2 poles (61.2081, -94.3365) (61.3108, -94.2959) (61.4051, -94.2959) knots 0 0 0 1 1 1
  line L141 (61.4051, -94.2959) -> (64.4759, -94.2959)
  line L142 (64.4759, -94.2959) -> (64.4759, -95.4694)
  spline S101 degree 2 poles (86.7727, -90.3561) (86.7727, -90.9599) (86.338, -91.4139) knots 0 0 0 1 1 1
  spline S102 degree 2 poles (86.338, -91.4139) (85.8605, -91.8529) (85.1987, -91.8529) knots 0 0 0 1 1 1
  line L143 (85.1987, -91.8529) -> (82.8153, -91.8529)
  line L144 (82.8153, -91.8529) -> (82.8153, -91.8122)
  spline S103 degree 2 poles (82.8153, -91.8122) (82.8153, -91.5103) (83.083, -91.2426) knots 0 0 0 1 1 1
  spline S104 degree 2 poles (83.083, -91.2426) (83.1622, -91.1741) (83.2372, -91.1313) knots 0 0 0 1 1 1
  spline S105 degree 2 poles (83.2372, -91.1313) (83.3121, -91.0884) (83.3892, -91.0649) knots 0 0 0 1 1 1
  spline S106 degree 2 poles (83.3892, -91.0649) (83.4663, -91.0435) (83.5498, -91.0349) knots 0 0 0 1 1 1
  spline S107 degree 2 poles (83.5498, -91.0349) (83.6333, -91.0285) (83.734, -91.0285) knots 0 0 0 1 1 1
  line L145 (83.734, -91.0285) -> (85.1816, -91.0285)
  spline S108 degree 2 poles (85.1816, -91.0285) (85.6335, -91.0285) (85.8091, -90.6023) knots 0 0 0 1 1 1
  spline S109 degree 2 poles (85.8091, -90.6023) (85.854, -90.4738) (85.854, -90.3239) knots 0 0 0 1 1 1
  line L146 (85.854, -90.3239) -> (85.854, -90.3068)
  spline S110 degree 2 poles (85.854, -90.3068) (85.854, -89.7543) (85.3379, -89.6194) knots 0 0 0 1 1 1
  spline S111 degree 2 poles (85.3379, -89.6194) (85.2309, -89.6065) (85.1816, -89.6065) knots 0 0 0 1 1 1
  line L147 (85.1816, -89.6065) -> (82.8153, -89.6065)
  line L148 (82.8153, -89.6065) -> (82.8153, -89.5616)
  spline S112 degree 2 poles (82.8153, -89.5616) (82.8153, -89.2489) (83.1066, -88.9705) knots 0 0 0 1 1 1
  spline S113 degree 2 poles (83.1066, -88.9705) (83.3592, -88.7821) (83.5948, -88.7821) knots 0 0 0 1 1 1
  line L149 (83.5948, -88.7821) -> (85.203, -88.7821)
  spline S114 degree 2 poles (85.203, -88.7821) (85.7791, -88.7821) (86.2352, -89.1226) knots 0 0 0 1 1 1
  spline S115 degree 2 poles (86.2352, -89.1226) (86.7727, -89.583) (86.7727, -90.2661) knots 0 0 0 1 1 1
  line L150 (86.7727, -90.2661) -> (86.7727, -90.3561)
  spline S116 degree 2 poles (82.1729, -91.5124) (82.1729, -91.7351) (81.9266, -91.8401) knots 0 0 0 1 1 1
  spline S117 degree 2 poles (81.9266, -91.8401) (81.8774, -91.8529) (81.8324, -91.8529) knots 0 0 0 1 1 1
  line L151 (81.8324, -91.8529) -> (81.2585, -91.8529)
  line L152 (81.2585, -91.8529) -> (81.2585, -88.7821)
  line L153 (81.2585, -88.7821) -> (82.1729, -88.7821)
  line L154 (82.1729, -88.7821) -> (82.1729, -91.5124)
  spline S118 degree 2 poles (80.616, -89.9556) (80.616, -90.1676) (80.4554, -90.401) knots 0 0 0 1 1 1
  spline S119 degree 2 poles (80.4554, -90.401) (80.2006, -90.7329) (79.7637, -90.7329) knots 0 0 0 1 1 1
  line L155 (79.7637, -90.7329) -> (79.6974, -90.7329)
  line L156 (79.6974, -90.7329) -> (79.6974, -90.2832)
  line L157 (79.6974, -90.2832) -> (77.9542, -90.2832)
  spline S120 degree 2 poles (77.9542, -90.2832) (77.7872, -90.2832) (77.6865, -90.371) knots 0 0 0 1 1 1
  spline S121 degree 2 poles (77.6865, -90.371) (77.5859, -90.461) (77.5859, -90.628) knots 0 0 0 1 1 1
  line L158 (77.5859, -90.628) -> (77.5859, -90.688)
  spline S122 degree 2 poles (77.5859, -90.688) (77.5859, -90.9385) (77.8193, -91.0156) knots 0 0 0 1 1 1
  spline S123 degree 2 poles (77.8193, -91.0156) (77.8514, -91.0285) (77.9092, -91.0285) knots 0 0 0 1 1 1
  line L159 (77.9092, -91.0285) -> (79.6974, -91.0285)
  spline S124 degree 2 poles (79.6974, -91.0285) (80.0657, -91.0285) (80.2391, -91.1634) knots 0 0 0 1 1 1
  spline S125 degree 2 poles (80.2391, -91.1634) (80.3205, -91.2126) (80.3912, -91.2833) knots 0 0 0 1 1 1
  spline S126 degree 2 poles (80.3912, -91.2833) (80.4597, -91.3561) (80.5111, -91.4439) knots 0 0 0 1 1 1
  spline S127 degree 2 poles (80.5111, -91.4439) (80.5604, -91.5339) (80.5882, -91.6366) knots 0 0 0 1 1 1
  spline S128 degree 2 poles (80.5882, -91.6366) (80.616, -91.7416) (80.616, -91.8529) knots 0 0 0 1 1 1
  line L160 (80.616, -91.8529) -> (77.8985, -91.8529)
  spline S129 degree 2 poles (77.8985, -91.8529) (77.6351, -91.8529) (77.4103, -91.7694) knots 0 0 0 1 1 1
  spline S130 degree 2 poles (77.4103, -91.7694) (77.1833, -91.6859) (77.0184, -91.5296) knots 0 0 0 1 1 1
  spline S131 degree 2 poles (77.0184, -91.5296) (76.8514, -91.3732) (76.7571, -91.1484) knots 0 0 0 1 1 1
  spline S132 degree 2 poles (76.7571, -91.1484) (76.6629, -90.9235) (76.6629, -90.643) knots 0 0 0 1 1 1
  spline S133 degree 2 poles (76.6629, -90.643) (76.6629, -90.0027) (77.1961, -89.6515) knots 0 0 0 1 1 1
  line L161 (77.1961, -89.6515) -> (77.2004, -89.6515)
  line L162 (77.2004, -89.6515) -> (77.2004, -89.6472)
  line L163 (77.2004, -89.6472) -> (76.3717, -88.7864)
  line L164 (76.3717, -88.7864) -> (76.3717, -88.7821)
  line L165 (76.3717, -88.7821) -> (77.5859, -88.7821)
  line L166 (77.5859, -88.7821) -> (78.2455, -89.4588)
  line L167 (78.2455, -89.4588) -> (79.6974, -89.4588)
  line L168 (79.6974, -89.4588) -> (79.6974, -88.7842)
  line L169 (79.6974, -88.7842) -> (80.616, -88.7842)
  line L170 (80.616, -88.7842) -> (80.616, -89.9556)
  spline S134 degree 2 poles (76.0505, -90.3561) (76.0505, -90.9599) (75.6157, -91.4139) knots 0 0 0 1 1 1
  spline S135 degree 2 poles (75.6157, -91.4139) (75.1382, -91.8529) (74.4765, -91.8529) knots 0 0 0 1 1 1
  line L171 (74.4765, -91.8529) -> (72.0931, -91.8529)
  line L172 (72.0931, -91.8529) -> (72.0931, -91.8122)
  spline S136 degree 2 poles (72.0931, -91.8122) (72.0931, -91.5103) (72.3607, -91.2426) knots 0 0 0 1 1 1
  spline S137 degree 2 poles (72.3607, -91.2426) (72.44, -91.1741) (72.5149, -91.1313) knots 0 0 0 1 1 1
  spline S138 degree 2 poles (72.5149, -91.1313) (72.5899, -91.0884) (72.667, -91.0649) knots 0 0 0 1 1 1
  spline S139 degree 2 poles (72.667, -91.0649) (72.7441, -91.0435) (72.8276, -91.0349) knots 0 0 0 1 1 1
  spline S140 degree 2 poles (72.8276, -91.0349) (72.9111, -91.0285) (73.0117, -91.0285) knots 0 0 0 1 1 1
  line L173 (73.0117, -91.0285) -> (74.4594, -91.0285)
  spline S141 degree 2 poles (74.4594, -91.0285) (74.9112, -91.0285) (75.0868, -90.6023) knots 0 0 0 1 1 1
  spline S142 degree 2 poles (75.0868, -90.6023) (75.1318, -90.4738) (75.1318, -90.3239) knots 0 0 0 1 1 1
  line L174 (75.1318, -90.3239) -> (75.1318, -90.3068)
  spline S143 degree 2 poles (75.1318, -90.3068) (75.1318, -89.7543) (74.6157, -89.6194) knots 0 0 0 1 1 1
  spline S144 degree 2 poles (74.6157, -89.6194) (74.5086, -89.6065) (74.4594, -89.6065) knots 0 0 0 1 1 1
  line L175 (74.4594, -89.6065) -> (72.0931, -89.6065)
  line L176 (72.0931, -89.6065) -> (72.0931, -89.5616)
  spline S145 degree 2 poles (72.0931, -89.5616) (72.0931, -89.2489) (72.3843, -88.9705) knots 0 0 0 1 1 1
  spline S146 degree 2 poles (72.3843, -88.9705) (72.637, -88.7821) (72.8725, -88.7821) knots 0 0 0 1 1 1
  line L177 (72.8725, -88.7821) -> (74.4808, -88.7821)
  spline S147 degree 2 poles (74.4808, -88.7821) (75.0568, -88.7821) (75.513, -89.1226) knots 0 0 0 1 1 1
  spline S148 degree 2 poles (75.513, -89.1226) (76.0505, -89.583) (76.0505, -90.2661) knots 0 0 0 1 1 1
  line L178 (76.0505, -90.2661) -> (76.0505, -90.3561)
  spline S149 degree 2 poles (71.4506, -91.4739) (71.4506, -91.718) (71.1765, -91.8379) knots 0 0 0 1 1 1
  spline S150 degree 2 poles (71.1765, -91.8379) (71.1294, -91.8529) (71.0716, -91.8529) knots 0 0 0 1 1 1
  line L179 (71.0716, -91.8529) -> (70.5555, -91.8529)
  line L180 (70.5555, -91.8529) -> (70.5555, -90.3239)
  spline S151 degree 2 poles (70.5555, -90.3239) (70.5555, -90.1912) (70.5148, -90.0841) knots 0 0 0 1 1 1
  spline S152 degree 2 poles (70.5148, -90.0841) (70.472, -89.977) (70.4013, -89.8956) knots 0 0 0 1 1 1
  spline S153 degree 2 poles (70.4013, -89.8956) (70.3285, -89.8143) (70.2321, -89.7543) knots 0 0 0 1 1 1
  spline S154 degree 2 poles (70.2321, -89.7543) (70.1336, -89.6965) (70.0244, -89.6579) knots 0 0 0 1 1 1
  spline S155 degree 2 poles (70.0244, -89.6579) (69.9131, -89.6215) (69.7953, -89.6044) knots 0 0 0 1 1 1
  spline S156 degree 2 poles (69.7953, -89.6044) (69.6775, -89.5873) (69.564, -89.5873) knots 0 0 0 1 1 1
  spline S157 degree 2 poles (69.564, -89.5873) (69.0993, -89.5873) (68.7524, -89.8378) knots 0 0 0 1 1 1
  spline S158 degree 2 poles (68.7524, -89.8378) (68.5125, -90.0434) (68.5125, -90.2961) knots 0 0 0 1 1 1
  line L181 (68.5125, -90.2961) -> (68.5125, -91.3561)
  spline S159 degree 2 poles (68.5125, -91.3561) (68.5125, -91.6217) (68.3948, -91.7202) knots 0 0 0 1 1 1
  spline S160 degree 2 poles (68.3948, -91.7202) (68.277, -91.8379) (68.1057, -91.8379) knots 0 0 0 1 1 1
  line L182 (68.1057, -91.8379) -> (67.5981, -91.8379)
  line L183 (67.5981, -91.8379) -> (67.5981, -90.2404)
  spline S161 degree 2 poles (67.5981, -90.2404) (67.5981, -89.5552) (68.2363, -89.1162) knots 0 0 0 1 1 1
  spline S162 degree 2 poles (68.2363, -89.1162) (68.7909, -88.7821) (69.4355, -88.7821) knots 0 0 0 1 1 1
  line L184 (69.4355, -88.7821) -> (69.5447, -88.7821)
  spline S163 degree 2 poles (69.5447, -88.7821) (70.2964, -88.7821) (70.9046, -89.204) knots 0 0 0 1 1 1
  spline S164 degree 2 poles (70.9046, -89.204) (71.4506, -89.6451) (71.4506, -90.2361) knots 0 0 0 1 1 1
  line L185 (71.4506, -90.2361) -> (71.4506, -91.4739)
  spline S165 degree 2 poles (66.9557, -91.5124) (66.9557, -91.7351) (66.7094, -91.8401) knots 0 0 0 1 1 1
  spline S166 degree 2 poles (66.7094, -91.8401) (66.6602, -91.8529) (66.6152, -91.8529) knots 0 0 0 1 1 1
  line L186 (66.6152, -91.8529) -> (66.0413, -91.8529)
  line L187 (66.0413, -91.8529) -> (66.0413, -88.7821)
  line L188 (66.0413, -88.7821) -> (66.9557, -88.7821)
  line L189 (66.9557, -88.7821) -> (66.9557, -91.5124)
  line L190 (64.0883, -91.0285) -> (65.5059, -91.0285)
  line L191 (65.5059, -91.0285) -> (65.5059, -91.1591)
  spline S167 degree 2 poles (65.5059, -91.1591) (65.5059, -91.384) (65.3089, -91.6195) knots 0 0 0 1 1 1
  spline S168 degree 2 poles (65.3089, -91.6195) (65.1269, -91.7887) (65.0091, -91.8122) knots 0 0 0 1 1 1
  spline S169 degree 2 poles (65.0091, -91.8122) (64.9021, -91.8529) (64.8121, -91.8529) knots 0 0 0 1 1 1
  line L192 (64.8121, -91.8529) -> (61.7413, -91.8529)
  line L193 (61.7413, -91.8529) -> (61.7413, -91.7266)
  spline S170 degree 2 poles (61.7413, -91.7266) (61.7413, -91.4996) (61.934, -91.2705) knots 0 0 0 1 1 1
  spline S171 degree 2 poles (61.934, -91.2705) (62.131, -91.0285) (62.57, -91.0285) knots 0 0 0 1 1 1
  line L194 (62.57, -91.0285) -> (63.1653, -91.0285)
  line L195 (63.1653, -91.0285) -> (63.1653, -88.7821)
  line L196 (63.1653, -88.7821) -> (64.0883, -88.7821)
  line L197 (64.0883, -88.7821) -> (64.0883, -91.0285)
extrude "Extrude14" cut sketch "Sketch9" against normal blind 1 contours L82 S3 S4 S5 S6 L83 S7 L84 S8 S9 S10 S11 S12 S17 S18 bodies 2 1
extrude "Extrude15" cut sketch "Sketch9" against normal blind 0.5 contours S0 S1 S2 L77 L78 L79 L80 L81 S12 S13 S14 S15 S16 | L85 S19 L86 L87 S20 S21 L88 L89 L90 S22 S23 S24 S25 S26 L91 L92 L93 L94 | S27 S28 S29 S30 L95 L96 L97 S31 S32 S33 S34 S35 S36 S37 S38 S39 S40 S41 S42 S43 S44 S45 S46 L98 L99 L100 | L101 L102 S47 S48 S49 L103 L104 S50 S51 L105 L106 L107 L108 | S52 S53 L109 L110 S54 S55 S56 S57 S58 S59 S60 S61 L111 S62 S63 L112 L113 S64 S65 L114 S66 S67 L115 | S68 S69 L116 L117 L118 S70 S71 L119 S72 S73 L120 S74 S75 S76 S77 S78 L121 S79 S80 S81 S82 S83 L122 L123 L124 L125 L126 L127 L128 L129 L130 L131 | S84 S85 S86 L132 L133 S87 S88 S89 S90 S91 L134 L135 | S92 S93 L136 S94 S95 S96 S97 L137 L138 L139 L140 S98 S99 S100 L141 L142 | S101 S102 L143 L144 S103 S104 S105 S106 S107 L145 S108 S109 L146 S110 S111 L147 L148 S112 S113 L149 S114 S115 L150 | S116 S117 L151 L152 L153 L154 | S118 S119 L155 L156 L157 S120 S121 L158 S122 S123 L159 S124 S125 S126 S127 S128 L160 S129 S130 S131 S132 S133 L161 L162 L163 L164 L165 L166 L167 L168 L169 L170 | S134 S135 L171 L172 S136 S137 S138 S139 S140 L173 S141 S142 L174 S143 S144 L175 L176 S145 S146 L177 S147 S148 L178 | S149 S150 L179 L180 S151 S152 S153 S154 S155 S156 S157 S158 L181 S159 S160 L182 L183 S161 S162 L184 S163 S164 L185 | S165 S166 L186 L187 L188 L189 | L190 L191 S167 S168 S169 L192 L193 S170 S171 L194 L195 L196 L197 bodies 2 1
sketch "Sketch10" plane through (102, 0, 0) normal (1, 0, 0) x (0, 1, 0)
  line L0 (2, 0) -> (102, 0)
  line L1 (102, 0) -> (102, 6.5)
  line L2 (23.85, 3) -> (25.85, 3)
  line L3 (25.85, 3) -> (25.85, 29)
  line L4 (25.85, 29) -> (23.85, 29)
  line L5 (23.85, 29) -> (23.85, 3)
  line L6 (23.85, 29) -> (25.85, 29)
  line L7 (25.85, 29) -> (25.85, 3)
  line L8 (25.85, 3) -> (23.85, 3)
  line L9 (23.85, 3) -> (23.85, 29)
  dimension "d135" = 21.85
  constraint horizontal L2
  constraint vertical L3
  constraint horizontal L4
  constraint vertical L5
  constraint horizontal L6
  constraint vertical L7
  constraint horizontal L8
  constraint vertical L9
  measures "d135" horizontal distance of L0.start L2.start
extrude "Extrude17" cut sketch "Sketch10" against normal blind 105 bodies 2
pattern_linear "R-Pattern4" count 12 spacing 5.9091 along (0, 1, 0) of "Extrude17"
move_body "Move1" bodies 2 to x (1, 0, 0) y (0, -1, 0) z (0, 0, -1) at (0, 104, 32.5)
named bodies: "bottom_box", "top_box", "solar_holder"
